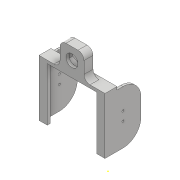
# Autodesk Inventor part: protoboard_harness
Saved by Autodesk Inventor 2017 (Build 210142000, 142)
## iProperties
Created: 2018-04-22
Part Number: protoboard_harness
Material: Generic
Document SubType Name: Modeling
Designer: mfans
Density: 1 g/cm^3
Appearance: Default
Author: mfans
Autodesk Inventor part; units mm, degrees
ref_plane "YZ Plane" through (0, 0, 0) normal (1, 0, 0) x (0, 1, 0)
ref_plane "XZ Plane" through (0, 0, 0) normal (0, 1, 0) x (-1, 0, 0)
ref_plane "XY Plane" through (0, 0, 0) normal (0, 0, 1) x (1, 0, 0)
sketch "Sketch1" plane through (0, 0, 0) normal (0, 1, 0) x (-1, 0, 0)
  line L0 (10.25, 22) -> (-10.25, 22)
  line L1 (-10.25, 22) -> (-10.25, -22)
  line L2 (-10.25, -22) -> (10.25, -22)
  line L3 (10.25, -22) -> (10.25, 22)
  line L4 (10.25, 22) -> (-10.25, -22) construction
  line L5 (-10.25, 22) -> (10.25, -22) construction
  line L6 (-11, 22) -> (11, 22)
  line L7 (11, 22) -> (11, -22)
  line L8 (11, -22) -> (-11, -22)
  line L9 (-11, -22) -> (-11, 22)
  line L10 (-11, 22) -> (11, -22) construction
  line L11 (11, 22) -> (-11, -22) construction
  point P0 (0, 0)
  dimension "d0" = 20.5
  dimension "d1" = 44
  dimension "d2" = 22
  constraints: 24 end point, 4 midpoint, 4 parallel, 2 horizontal, 2 perpendicular
  measures "d0" distance of L2.end L1.end
  measures "d1" distance of L0.end L1.end
  measures "d2" distance of L7.end L8.end
extrude "Extrusion1" add sketch "Sketch1" along normal blind 11 contours L6 L7 L8 L3 | L1 L8 L9 L6
sketch "Sketch2" plane through (-11, 0, 22) normal (0, 0, 1) x (1, 0, 0)
  line L0 (0.75, 0) -> (0.75, 11) projected
  line L1 (0.75, 0) -> (0.75, 11) projected
  line L2 (0, 11) -> (0.75, 11) projected
  line L3 (0, 0) -> (0, 11) projected
  line L4 (0.75, 0) -> (0, 0) projected
  line L5 (21.25, 11) -> (21.25, 0) projected
  line L6 (22, 0) -> (21.25, 0) projected
  line L7 (22, 0) -> (22, 11) projected
  line L8 (21.25, 11) -> (22, 11) projected
  line L9 (0, 0) -> (0, 11) projected
  line L10 (22, 0) -> (22, 11) projected
  line L11 (0, 0) -> (22, 0)
  line L12 (22, 0) -> (22, 3)
  line L13 (22, 3) -> (0, 3)
  line L14 (0, 3) -> (0, 0)
  point P0 (11, 0)
  dimension "d5" = 3
  constraints: 8 end point, 2 parallel, 1 horizontal, 1 perpendicular, 1 point on line
  measures "d5" distance between parallel lines of L11 L13
extrude "Extrusion2" add sketch "Sketch2" along normal blind 1 contours L4 L3 L13 L0 | L0 L13 L5 L11 | L5 L13 L7 L6
mirror "Mirror1" about plane through (0, 0, 0) normal (0, 0, 1) of "Extrusion2"
sketch "Sketch3" plane through (0, 0, 0) normal (0, -1, 0) x (1, 0, 0)
  line L0 (-11, -23) -> (11, -23) projected
  line L1 (8.25, -23) -> (11, -23)
  line L2 (11, -23) -> (11, 23)
  line L3 (11, 23) -> (8.25, 23)
  line L4 (8.25, 23) -> (8.25, -23)
  line L5 (10.25, 22) -> (10.25, -22) projected
  line L6 (-10.25, -22) -> (-10.25, 22) projected
  line L7 (-10.25, 22) -> (10.25, 22) projected
  line L8 (10.25, 22) -> (10.25, -22) projected
  line L9 (-10.25, -22) -> (10.25, -22) projected
  line L10 (-11, 23) -> (-11, -23) projected
  line L11 (-11, -23) -> (11, -23) projected
  line L12 (11, -23) -> (11, 23) projected
  line L13 (-11, 23) -> (11, 23) projected
  line L14 (-11, -23) -> (-8.25, -23)
  line L15 (-8.25, -23) -> (-8.25, 23)
  line L16 (-8.25, 23) -> (-11, 23)
  line L17 (-11, 23) -> (-11, -23)
  point P0 (0, 0)
  dimension "d9" = 2
  dimension "d10" = 2
  constraints: 16 end point, 4 parallel, 2 horizontal, 2 perpendicular, 2 point on line
  measures "d9" distance between parallel lines of L5 L4
  measures "d10" distance between parallel lines of L6 L15
extrude "Extrusion3" add sketch "Sketch3" along normal blind 1 contours L10 L13 L15 L7 L6 L9 L0 | L15 L9 L4 L0 | L4 L9 L5 L7 L3 L2 L0 | L9 L6 L7 L15 | L13 L4 L7 L15 | L4 L7 L5 L9
sketch "Sketch4" plane through (11, -1, 23) normal (1, 0, 0) x (0, 0, -1)
  line L0 (1, 4) -> (1, 12) projected
  line L1 (0, 4) -> (0, 0) projected
  line L2 (46, 0) -> (0, 0) projected
  line L3 (46, 0) -> (46, 4) projected
  line L4 (45, 4) -> (45, 12) projected
  line L5 (1, 12) -> (45, 12) projected
  line L6 (45.7791, 4) -> (18.7791, 4)
  line L7 (18.7791, 4) -> (18.7791, 20.689)
  line L8 (18.7791, 20.689) -> (45.7791, 20.689)
  line L9 (45.7791, 20.689) -> (45.7791, 4)
  line L10 (45, 4) -> (46, 4) projected
  line L11 (1, 4) -> (0, 4) projected
  point P0 (23, 1)
  dimension "d14" = 27
  constraints: 8 end point, 2 parallel, 1 horizontal, 1 perpendicular
  measures "d14" distance of L7.end L8.end
extrude "Extrusion4" cut sketch "Sketch4" against normal through all contours L7 L8 L9 L6 L4 L5 | L5 L4 L6 L7
sketch "Sketch5" plane through (11, -1, 23) normal (1, 0, 0) x (0, 0, -1)
  point P0 (23, 1)
sketch "Sketch6" plane through (11, -1, 23) normal (1, 0, 0) x (0, 0, -1)
  line L0 (46, 4) -> (18.7791, 4) projected
  line L1 (18.7791, 4) -> (18.7791, 12) projected
  line L2 (1, 12) -> (18.7791, 12) projected
  line L3 (1, 4) -> (1, 12) projected
  line L4 (0, 4) -> (0, 0) projected
  line L5 (46, 0) -> (0, 0) projected
  line L6 (46, 0) -> (46, 4) projected
  line L7 (18.7791, 8.8707) -> (57.7172, 8.8707)
  line L8 (57.7172, 8.8707) -> (57.7172, -3.4205)
  line L9 (57.7172, -3.4205) -> (18.7791, -3.4205)
  line L10 (18.7791, -3.4205) -> (18.7791, 8.8707)
  line L11 (1, 4) -> (0, 4) projected
  point P0 (23, 1)
  constraints: 8 end point, 2 parallel, 1 horizontal, 1 perpendicular, 1 point on line
extrude "Extrusion5" cut sketch "Sketch6" against normal through all contours L6 L5 L10 L0 | L0 L1 L7 L8 L9 L10 L5 L6
sketch "Sketch7" plane through (-11, 3, 22) normal (-1, 0, 0) x (0, 0, 1)
  line L0 (1, -4) -> (-17.7791, -4) projected
  line L1 (1, 0) -> (1, -4) projected
  point P0 (-22, -3)
  point P1 (-7, 2)
  point P2 (-10, 2)
  dimension "d19" = 6
  dimension "d20" = 6
  dimension "d21" = 8
  dimension "d22" = 3
  measures "d19" distance from line of L0 point (-7, 2)
  measures "d20" distance from line of L0 point (-10, 2)
  measures "d21" distance from line of L1 point (-7, 2)
  measures "d22" distance of point (-7, 2) point (-10, 2)
hole "Hole1" at (-11, 5, 15) at (-11, 5, 12) direction (1, 0, 0) diameter 0.7 end through all
sketch "Sketch8" plane through (0, -1, 0) normal (0, -1, 0) x (1, 0, 0)
  line L0 (-11, 4.2209) -> (-8.25, 4.2209) projected
  line L1 (-8.25, 22) -> (-8.25, 4.2209) projected
  line L2 (-8.25, 22) -> (8.25, 22) projected
  line L3 (8.25, 4.2209) -> (8.25, 22) projected
  line L4 (8.25, 4.2209) -> (11, 4.2209) projected
  line L5 (11, 4.2209) -> (11, 23) projected
  line L6 (11, 23) -> (-11, 23) projected
  line L7 (-11, 23) -> (-11, 4.2209) projected
  line L8 (11, 23) -> (-11, 23) projected
  line L9 (4, 31) -> (-4, 31)
  line L10 (-4, 31) -> (-4, 23)
  line L11 (-4, 23) -> (4, 23)
  line L12 (4, 23) -> (4, 31)
  line L13 (4, 31) -> (-4, 23) construction
  line L14 (-4, 31) -> (4, 23) construction
  point P0 (0, 0)
  point P1 (0, 27)
  dimension "d30" = 8
  dimension "d31" = 0
  dimension "d32" = 8
  constraints: 12 end point, 2 midpoint, 2 parallel, 1 horizontal, 1 perpendicular, 1 point on line
  measures "d30" distance of L9.start L9.end
  measures "d31" horizontal distance of point (0, 0) point (0, 27)
  measures "d32" distance of L9.end L10.end
extrude "Extrusion6" add sketch "Sketch8" against normal blind 3 contours L10 L9 L12 L6
sketch "Sketch9" plane through (-10.25, 3, 22) normal (0, 1, 0) x (1, 0, 0)
  line L0 (20.5, 0) -> (21.25, 0) projected
  line L1 (20.5, 0) -> (0, 0) projected
  line L2 (-0.75, 0) -> (0, 0) projected
  line L3 (-0.75, 0) -> (-0.75, -1) projected
  line L4 (21.25, -1) -> (-0.75, -1) projected
  line L5 (21.25, 0) -> (21.25, -1) projected
  line L6 (7.5011, -6.5896) -> (7.4989, -3.4141)
  line L7 (7.4989, -3.4141) -> (10.2478, -1.8246)
  line L8 (10.2478, -1.8246) -> (12.9989, -3.4104)
  line L9 (12.9989, -3.4104) -> (13.0011, -6.5859)
  line L10 (13.0011, -6.5859) -> (10.2522, -8.1754)
  line L11 (10.2522, -8.1754) -> (7.5011, -6.5896)
  line L12 (6.25, -1) -> (14.25, -1) projected
  line L13 (6.25, -1) -> (6.25, -9) projected
  line L14 (6.25, -9) -> (14.25, -9) projected
  line L15 (14.25, -9) -> (14.25, -1) projected
  point P0 (10.25, 22)
  point P1 (10.25, -5)
  dimension "d35" = 5.5
  dimension "d38" = 4
  constraints: 12 end point, 13 other
  measures "d35" distance between parallel lines of L9 L6
  measures "d38" distance from line of L14 point (10.25, -5)
extrude "Extrusion7" cut sketch "Sketch9" against normal blind 3 contours L6 L7 L8 L9 L10 L11
sketch "Sketch10" plane through (-10.25, 0, 22) normal (0, 1, 0) x (1, 0, 0)
  line L0 (7.5011, -6.5896) -> (7.4989, -3.4141) projected
  line L1 (10.2522, -8.1754) -> (7.5011, -6.5896) projected
  line L2 (13.0011, -6.5859) -> (10.2522, -8.1754) projected
  line L3 (12.9989, -3.4104) -> (13.0011, -6.5859) projected
  line L4 (10.2478, -1.8246) -> (12.9989, -3.4104) projected
  line L5 (7.4989, -3.4141) -> (10.2478, -1.8246) projected
  point P0 (10.25, 22)
  point P1 (10.2478, -4.9963)
hole "Hole2" at (-0.0022, 0, 26.9963) direction (0, -1, 0) diameter 4 end through all
fillet "Fillet3" radius 2 2 edges at (-4, 0.5, 31) (4, 0.5, 31)
fillet "Fillet4" radius 2 2 edges at (4, 0.5, 23) (-4, 0.5, 23)
fillet "Fillet5" radius 6 4 edges at (-10.625, 11, 22) (10.625, 11, 22) (10.625, 11, 4.2209) (-10.625, 11, 4.2209)
body "Solid1"
